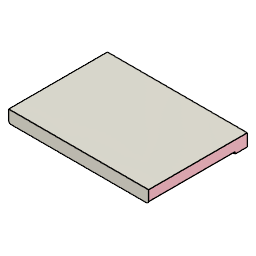
bottom_face_plate (Autodesk Fusion 360 design; units mm, degrees)
part number: 2025-10-08-20-58-30-384
Autodesk Fusion 360 part; units mm, degrees
sketch "Bottom Face Plate" plane through (0, 0, 0) normal (0, 0, 1) x (1, 0, 0)
  line L0 (0, 0) -> (136, 0)
  line L1 (136, 0) -> (136, 96)
  line L2 (136, 96) -> (0, 96)
  line L3 (0, 96) -> (0, 0)
  dimension "d5" = 136
  dimension "d6" = 96
  constraint horizontal L0
  constraint vertical L1
  constraint horizontal L2
  constraint vertical L3
  constraint coincident L0.start L3.end
  measures "d5" distance of L0.start L0.end
  measures "d6" distance of L0.start L2.end
extrude "Extrude1" add sketch "Bottom Face Plate" along normal blind 12 makes body 1
ref_plane "WorkPlane1" through (68, 84, 6) normal (0, 1, 0) x (-1, 0, 0)
split "Split1" by plane through (68, 84, 6) normal (0, 1, 0) bodies 1 makes body 2 at (90.6667, 96, 8)
fillet "Fillet1" radius 2 2 edges at (136, 42, 0) (0, 42, 0) on bodies 1
combine "Combine2" operation add target body 1 tool bodies 2
equation "block_size = 16 mm" comment "The size of the blocks used for the dimensions of the Minecraft Pig."
equation "pine_thickness = 12 mm" comment "The thickness of the pine boards used for the Minecraft Pig's body."
equation "bottom_face_plate_length = 6 * block_size" comment "The length of the Bottom Face Plate that makes up the Minecraft Pig's face."
equation "bottom_face_plate_width = 10 * block_size - 2 * pine_thickness" comment "The width of the Bottom Face Plate that makes up the Minecraft Pig's face."
equation "d5 = bottom_face_plate_width"
equation "d6 = bottom_face_plate_length"
equation "d7 = pine_thickness"
equation "d9 = -pine_thickness"
equation "fillet_radius = 2 mm" comment "The radius of the fillets applied to the Bottom Face Plate."
equation "d12 = fillet_radius"
named bodies: "Bottom Face Plate", "Bottom Face Plate (1)"
